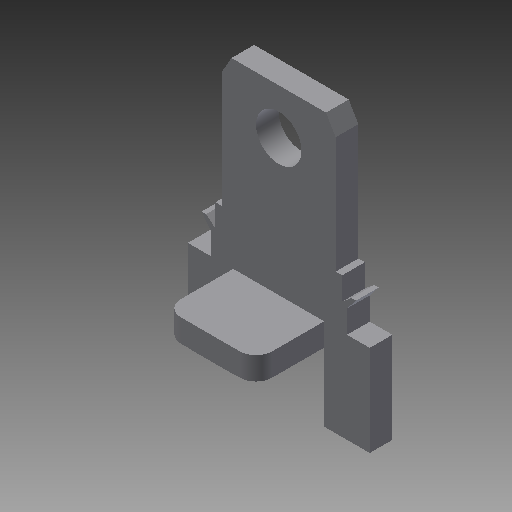
# Autodesk Inventor part: Pieza2
Saved by Autodesk Inventor 2019 (Build 230136000, 136)
## iProperties
Created: 2016-05-14
Part Number: Pieza2
Material: Genérico
Document SubType Name: Modeling
Designer: Isra
Density: 1 g/cm^3
Appearance: Valor por defecto
Author: Isra
Autodesk Inventor part; units mm, degrees
ref_plane "YZ Plane" through (0, 0, 0) normal (1, 0, 0) x (0, 1, 0)
ref_plane "XZ Plane" through (0, 0, 0) normal (0, 1, 0) x (-1, 0, 0)
ref_plane "XY Plane" through (0, 0, 0) normal (0, 0, 1) x (1, 0, 0)
sketch "Boceto1" plane through (0, 0, 0) normal (0, 0, 1) x (1, 0, 0)
  circle A0 centre (-5, 18) radius 1 projected
  line L0 (-8.3939, 13.4965) -> (-8, 13) projected
  line L1 (-8, 13) -> (-8, 12) projected
  line L2 (-2, 13) -> (-2, 12) projected
  line L3 (-2, 13) -> (-1.6061, 13.4965) projected
  line L4 (-1.6061, 13.4965) -> (-1.8061, 13.4965) projected
  line L5 (-1.8061, 13.4965) -> (-2.2146, 13.1547) projected
  line L6 (-2.2146, 13.1547) -> (-2.2146, 14.1547) projected
  line L7 (-2.2146, 14.1547) -> (-2.5, 14.1547) projected
  line L8 (-2.5, 14.1547) -> (-2.5, 19.2702) projected
  line L9 (-2.5, 19.2702) -> (-2.9213, 20) projected
  line L10 (-2.9213, 20) -> (-7.0787, 20) projected
  line L11 (-7.0787, 20) -> (-7.5, 19.2702) projected
  line L12 (-7.5, 19.2702) -> (-7.5, 14.1547) projected
  line L13 (-7.5, 14.1547) -> (-7.7854, 14.1547) projected
  line L14 (-7.7854, 14.1547) -> (-7.7854, 13.1547) projected
  line L15 (-7.7854, 13.1547) -> (-8.1939, 13.4965) projected
  line L16 (-8.1939, 13.4965) -> (-8.3939, 13.4965) projected
  line L17 (-8, 12) -> (-9, 12) projected
  line L18 (-9, 12) -> (-9, 8) projected
  line L19 (-7, 8) -> (-9, 8) projected
  line L20 (-7, 8) -> (-7, 11) projected
  line L21 (-3, 11) -> (-3, 8) projected
  line L22 (-1, 8) -> (-3, 8) projected
  line L23 (-1, 12) -> (-1, 8) projected
  line L24 (-1, 12) -> (-2, 12) projected
  line L25 (-3, 11) -> (-7, 11) projected
  point P0 (0, 0)
extrude "Extrusión1" add sketch "Boceto1" along normal blind 1
sketch "Boceto6" plane through (0, 0, 1) normal (0, 0, 1) x (1, 0, 0)
  line L0 (-3, 11) -> (-3, 8) projected
  line L1 (-7, 11) -> (-3, 11)
  line L2 (-3, 11) -> (-3, 10)
  line L3 (-3, 10) -> (-7, 10)
  line L4 (-7, 10) -> (-7, 11)
  point P0 (0, 0)
  point P1 (-3, 12)
  dimension "d19" = 1
  dimension "d20" = 4
  constraints: 8 end point, 2 parallel, 1 horizontal, 1 perpendicular, 1 point on line
  measures "d19" distance of L3.end L1.start
  measures "d20" distance of L1.start L0.start
sketch "Boceto7" plane through (-7, 12, 0) normal (0, -1, 0) x (1, 0, 0)
  line L0 (0, 0) -> (4, 0) projected
  line L1 (4, 0) -> (4, 1) projected
  line L2 (0, 1) -> (4, 1) projected
  line L3 (0, 0) -> (0, 1) projected
  line L4 (0, 0) -> (4, 0)
  line L5 (4, 0) -> (4, 1)
  line L6 (4, 1) -> (0, 1)
  line L7 (0, 1) -> (0, 0)
  point P0 (7, 0)
  constraints: 8 end point, 2 parallel, 1 horizontal, 1 perpendicular
feature "Barrido2" [suppressed]
fillet "Empalme4" [suppressed]
sketch "Boceto8" plane through (0, 0, 1) normal (0, 0, 1) x (1, 0, 0)
  line L0 (-3.001, 11.0119) -> (-7.001, 11.0119)
  line L1 (-7.001, 11.0119) -> (-7.001, 12.0119)
  line L2 (-7.001, 12.0119) -> (-3.001, 12.0119)
  line L3 (-3.001, 12.0119) -> (-3.001, 11.0119)
  point P0 (0, 0)
  dimension "d24" = 4
  dimension "d25" = 1
  constraints: 8 end point, 2 parallel, 1 horizontal, 1 perpendicular
  measures "d24" distance of L1.end L2.end
  measures "d25" distance of L0.end L1.end
extrude "Extrusión4" add sketch "Boceto8" along normal blind 3
fillet "Empalme5" radius 0.7 2 edges at (-7.001, 11.5119, 4) (-3.001, 11.5119, 4)
